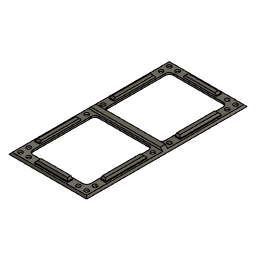
Frame Outer PLA Optimised v3 (Autodesk Fusion 360 design; units mm, degrees)
Autodesk Fusion 360 part; units mm, degrees
sketch "Sketch1" plane through (0, 0, 0) normal (0, 0, 1) x (1, 0, 0)
  line L0 (0, 0) -> (100, 0)
  line L1 (100, 0) -> (100, 200)
  line L2 (100, 200) -> (0, 200)
  line L3 (0, 200) -> (0, 0)
  line L4 (15, 15) -> (85, 15)
  line L5 (85, 15) -> (85, 185)
  line L6 (85, 185) -> (15, 185)
  line L7 (15, 185) -> (15, 15)
  dimension "d1" = 100
  dimension "d2" = 200
  dimension "d5" = 70
  dimension "d6" = 170
  dimension "d7" = 70
  constraint horizontal L0
  constraint vertical L1
  constraint horizontal L2
  constraint vertical L3
  constraint coincident L0.start L3.end
  constraint perpendicular L1 L4
  constraint perpendicular L2 L5
  constraint perpendicular L5 L6
  measures "d1" distance of L0.start L0.end
  measures "d2" distance of L0.start L2.end
  measures "d5" distance of L4.start L4.end
  measures "d6" distance of L4.end L5.end
  measures "d7" distance of L5.end L6.end
extrude "Extrude1" add sketch "Sketch1" along normal blind 5
fillet "Fillet1" radius 5 1 edges at (15, 185, 2.5)
fillet "Fillet2" radius 5 1 edges at (85, 185, 2.5)
fillet "Fillet3" radius 5 1 edges at (85, 15, 2.5)
fillet "Fillet4" radius 5 1 edges at (15, 15, 2.5)
chamfer "Chamfer1" distance 5 angle 45 1 edges at (0, 100, 5)
chamfer "Chamfer2" distance 5 angle 45 1 edges at (100, 100, 5)
chamfer "Chamfer3" distance 5 angle 45 1 edges at (50, 0, 5)
chamfer "Chamfer4" distance 5 angle 45 1 edges at (50, 200, 5)
sketch "Sketch2" plane through (0, 0, 5) normal (0, 0, 1) x (-1, 0, 0)
  line L0 (-15, -20) -> (-15, -180)
  arc A0 (-20, -185) -> (-15, -180) centre (-20, -180) ccw
  line L1 (-20, -185) -> (-80, -185)
  arc A1 (-85, -180) -> (-80, -185) centre (-80, -180) ccw
  line L2 (-85, -180) -> (-85, -20)
  arc A2 (-80, -15) -> (-85, -20) centre (-80, -20) ccw
  line L3 (-80, -15) -> (-20, -15)
  arc A3 (-15, -20) -> (-20, -15) centre (-20, -20) ccw
  line L4 (-95, -195) -> (-5, -195)
  line L5 (-5, -195) -> (-5, -5)
  line L6 (-5, -5) -> (-95, -5)
  line L7 (-95, -5) -> (-95, -195)
  line L8 (-95, -5) -> (-95, -100)
  line L9 (-95, -100) -> (-90, -100)
  line L10 (-90, -100) -> (-5, -100)
  line L11 (-85, -100) -> (-85, -105)
  line L12 (-85, -100) -> (-85, -95)
  line L13 (-85, -105) -> (-77.8443, -105)
  line L14 (-77.8443, -105) -> (-15, -105)
  line L15 (-85, -95) -> (-15, -95)
  dimension "d22" = 95
  dimension "d23" = 5
  constraint coincident L6.end L7.start
  constraint perpendicular L6 L8
  constraint perpendicular L7 L9
  constraint midpoint L5 L10.end
  constraint perpendicular L5 L10
  constraint midpoint L2 L11.start
  constraint perpendicular L10 L11
  constraint coincident L2 L12.end
  constraint perpendicular L10 L12
  constraint perpendicular L11 L13
  constraint coincident L0 L14.end
  constraint perpendicular L0 L14
  constraint coincident L0 L15.end
  constraint perpendicular L0 L15
  measures "d22" distance of L6.end L8.end
  measures "d23" distance of L11.start L11.end
extrude "Extrude2" add sketch "Sketch2" against normal blind 5 contours L0 L2 L10 L12 L15 | L0 L2 L10 L11 L13 L14
fillet "Fillet5" radius 5 1 edges at (85, 105, 2.5)
fillet "Fillet6" radius 5 1 edges at (15, 105, 2.5)
fillet "Fillet7" radius 5 1 edges at (15, 95, 2.5)
fillet "Fillet8" radius 5 1 edges at (85, 95, 2.5)
sketch "Sketch3" plane through (0, 0, 5) normal (0, 0, 1) x (-1, 0, 0)
  line L0 (-15, -110) -> (-15, -180)
  arc A0 (-20, -185) -> (-15, -180) centre (-20, -180) ccw
  line L1 (-20, -185) -> (-80, -185)
  arc A1 (-85, -180) -> (-80, -185) centre (-80, -180) ccw
  line L2 (-85, -180) -> (-85, -110)
  arc A2 (-80, -105) -> (-85, -110) centre (-80, -110) ccw
  line L3 (-80, -105) -> (-20, -105)
  arc A3 (-15, -110) -> (-20, -105) centre (-20, -110) ccw
  line L4 (-85, -90) -> (-85, -20)
  arc A4 (-80, -15) -> (-85, -20) centre (-80, -20) ccw
  line L5 (-80, -15) -> (-20, -15)
  arc A5 (-15, -20) -> (-20, -15) centre (-20, -20) ccw
  line L6 (-15, -20) -> (-15, -90)
  arc A6 (-20, -95) -> (-15, -90) centre (-20, -90) ccw
  line L7 (-20, -95) -> (-80, -95)
  arc A7 (-85, -90) -> (-80, -95) centre (-80, -90) ccw
  line L8 (-95, -195) -> (-5, -195)
  line L9 (-5, -195) -> (-5, -5)
  line L10 (-5, -5) -> (-95, -5)
  line L11 (-95, -5) -> (-95, -195)
  circle A8 centre (-10, -10) radius 2.5
  dimension "d34" = 5
  measures "d34" diameter of A8
extrude "Extrude3" cut sketch "Sketch3" against normal blind 5 contours A8
sketch "Sketch4" plane through (0, 0, 5) normal (0, 0, 1) x (-1, 0, 0)
  circle A0 centre (-10, -10) radius 2.5
  line L0 (-15, -110) -> (-15, -180)
  arc A1 (-20, -185) -> (-15, -180) centre (-20, -180) ccw
  line L1 (-20, -185) -> (-80, -185)
  arc A2 (-85, -180) -> (-80, -185) centre (-80, -180) ccw
  line L2 (-85, -180) -> (-85, -110)
  arc A3 (-80, -105) -> (-85, -110) centre (-80, -110) ccw
  line L3 (-80, -105) -> (-20, -105)
  arc A4 (-15, -110) -> (-20, -105) centre (-20, -110) ccw
  line L4 (-85, -90) -> (-85, -20)
  arc A5 (-80, -15) -> (-85, -20) centre (-80, -20) ccw
  line L5 (-80, -15) -> (-20, -15)
  arc A6 (-15, -20) -> (-20, -15) centre (-20, -20) ccw
  line L6 (-15, -20) -> (-15, -90)
  arc A7 (-20, -95) -> (-15, -90) centre (-20, -90) ccw
  line L7 (-20, -95) -> (-80, -95)
  arc A8 (-85, -90) -> (-80, -95) centre (-80, -90) ccw
  line L8 (-95, -195) -> (-5, -195)
  line L9 (-5, -195) -> (-5, -5)
  line L10 (-5, -5) -> (-95, -5)
  line L11 (-95, -5) -> (-95, -195)
  circle A9 centre (-90, -10) radius 2.5
  dimension "d37" = 5
  measures "d37" diameter of A9
extrude "Extrude4" cut sketch "Sketch4" against normal blind 5 contours A9
sketch "Sketch5" plane through (0, 0, 5) normal (0, 0, 1) x (-1, 0, 0)
  circle A0 centre (-90, -10) radius 2.5
  circle A1 centre (-10, -10) radius 2.5
  line L0 (-15, -110) -> (-15, -180)
  arc A2 (-20, -185) -> (-15, -180) centre (-20, -180) ccw
  line L1 (-20, -185) -> (-80, -185)
  arc A3 (-85, -180) -> (-80, -185) centre (-80, -180) ccw
  line L2 (-85, -180) -> (-85, -110)
  arc A4 (-80, -105) -> (-85, -110) centre (-80, -110) ccw
  line L3 (-80, -105) -> (-20, -105)
  arc A5 (-15, -110) -> (-20, -105) centre (-20, -110) ccw
  line L4 (-85, -90) -> (-85, -20)
  arc A6 (-80, -15) -> (-85, -20) centre (-80, -20) ccw
  line L5 (-80, -15) -> (-20, -15)
  arc A7 (-15, -20) -> (-20, -15) centre (-20, -20) ccw
  line L6 (-15, -20) -> (-15, -90)
  arc A8 (-20, -95) -> (-15, -90) centre (-20, -90) ccw
  line L7 (-20, -95) -> (-80, -95)
  arc A9 (-85, -90) -> (-80, -95) centre (-80, -90) ccw
  line L8 (-95, -195) -> (-5, -195)
  line L9 (-5, -195) -> (-5, -5)
  line L10 (-5, -5) -> (-95, -5)
  line L11 (-95, -5) -> (-95, -195)
  circle A10 centre (-90, -190) radius 2.5
  dimension "d40" = 5
  measures "d40" diameter of A10
extrude "Extrude5" cut sketch "Sketch5" against normal blind 5 contours A10
sketch "Sketch6" plane through (0, 0, 5) normal (0, 0, 1) x (-1, 0, 0)
  circle A0 centre (-90, -190) radius 2.5
  circle A1 centre (-90, -10) radius 2.5
  circle A2 centre (-10, -10) radius 2.5
  line L0 (-15, -110) -> (-15, -180)
  arc A3 (-20, -185) -> (-15, -180) centre (-20, -180) ccw
  line L1 (-20, -185) -> (-80, -185)
  arc A4 (-85, -180) -> (-80, -185) centre (-80, -180) ccw
  line L2 (-85, -180) -> (-85, -110)
  arc A5 (-80, -105) -> (-85, -110) centre (-80, -110) ccw
  line L3 (-80, -105) -> (-20, -105)
  arc A6 (-15, -110) -> (-20, -105) centre (-20, -110) ccw
  line L4 (-85, -90) -> (-85, -20)
  arc A7 (-80, -15) -> (-85, -20) centre (-80, -20) ccw
  line L5 (-80, -15) -> (-20, -15)
  arc A8 (-15, -20) -> (-20, -15) centre (-20, -20) ccw
  line L6 (-15, -20) -> (-15, -90)
  arc A9 (-20, -95) -> (-15, -90) centre (-20, -90) ccw
  line L7 (-20, -95) -> (-80, -95)
  arc A10 (-85, -90) -> (-80, -95) centre (-80, -90) ccw
  line L8 (-95, -195) -> (-5, -195)
  line L9 (-5, -195) -> (-5, -5)
  line L10 (-5, -5) -> (-95, -5)
  line L11 (-95, -5) -> (-95, -195)
  circle A11 centre (-10, -190) radius 2.5
  dimension "d43" = 5
  measures "d43" diameter of A11
extrude "Extrude6" cut sketch "Sketch6" against normal blind 5 contours A11
sketch "Sketch7" plane through (0, 0, 5) normal (0, 0, 1) x (-1, 0, 0)
  circle A0 centre (-10, -190) radius 2.5
  circle A1 centre (-90, -190) radius 2.5
  circle A2 centre (-90, -10) radius 2.5
  circle A3 centre (-10, -10) radius 2.5
  line L0 (-15, -110) -> (-15, -180)
  arc A4 (-20, -185) -> (-15, -180) centre (-20, -180) ccw
  line L1 (-20, -185) -> (-80, -185)
  arc A5 (-85, -180) -> (-80, -185) centre (-80, -180) ccw
  line L2 (-85, -180) -> (-85, -110)
  arc A6 (-80, -105) -> (-85, -110) centre (-80, -110) ccw
  line L3 (-80, -105) -> (-20, -105)
  arc A7 (-15, -110) -> (-20, -105) centre (-20, -110) ccw
  line L4 (-85, -90) -> (-85, -20)
  arc A8 (-80, -15) -> (-85, -20) centre (-80, -20) ccw
  line L5 (-80, -15) -> (-20, -15)
  arc A9 (-15, -20) -> (-20, -15) centre (-20, -20) ccw
  line L6 (-15, -20) -> (-15, -90)
  arc A10 (-20, -95) -> (-15, -90) centre (-20, -90) ccw
  line L7 (-20, -95) -> (-80, -95)
  arc A11 (-85, -90) -> (-80, -95) centre (-80, -90) ccw
  line L8 (-95, -195) -> (-5, -195)
  line L9 (-5, -195) -> (-5, -5)
  line L10 (-5, -5) -> (-95, -5)
  line L11 (-95, -5) -> (-95, -195)
  circle A12 centre (-90, -90) radius 2.5
  dimension "d46" = 5
  measures "d46" diameter of A12
extrude "Extrude7" cut sketch "Sketch7" against normal blind 5 contours A12
sketch "Sketch8" plane through (0, 0, 5) normal (0, 0, 1) x (-1, 0, 0)
  circle A0 centre (-90, -90) radius 2.5
  circle A1 centre (-10, -190) radius 2.5
  circle A2 centre (-90, -190) radius 2.5
  circle A3 centre (-90, -10) radius 2.5
  circle A4 centre (-10, -10) radius 2.5
  line L0 (-15, -110) -> (-15, -180)
  arc A5 (-20, -185) -> (-15, -180) centre (-20, -180) ccw
  line L1 (-20, -185) -> (-80, -185)
  arc A6 (-85, -180) -> (-80, -185) centre (-80, -180) ccw
  line L2 (-85, -180) -> (-85, -110)
  arc A7 (-80, -105) -> (-85, -110) centre (-80, -110) ccw
  line L3 (-80, -105) -> (-20, -105)
  arc A8 (-15, -110) -> (-20, -105) centre (-20, -110) ccw
  line L4 (-85, -90) -> (-85, -20)
  arc A9 (-80, -15) -> (-85, -20) centre (-80, -20) ccw
  line L5 (-80, -15) -> (-20, -15)
  arc A10 (-15, -20) -> (-20, -15) centre (-20, -20) ccw
  line L6 (-15, -20) -> (-15, -90)
  arc A11 (-20, -95) -> (-15, -90) centre (-20, -90) ccw
  line L7 (-20, -95) -> (-80, -95)
  arc A12 (-85, -90) -> (-80, -95) centre (-80, -90) ccw
  line L8 (-95, -195) -> (-5, -195)
  line L9 (-5, -195) -> (-5, -5)
  line L10 (-5, -5) -> (-95, -5)
  line L11 (-95, -5) -> (-95, -195)
  circle A13 centre (-90, -110) radius 2.5
  dimension "d49" = 5
  measures "d49" diameter of A13
extrude "Extrude8" cut sketch "Sketch8" against normal blind 5 contours A13
sketch "Sketch9" plane through (0, 0, 5) normal (0, 0, 1) x (-1, 0, 0)
  circle A0 centre (-90, -110) radius 2.5
  circle A1 centre (-90, -90) radius 2.5
  circle A2 centre (-10, -190) radius 2.5
  circle A3 centre (-90, -190) radius 2.5
  circle A4 centre (-90, -10) radius 2.5
  circle A5 centre (-10, -10) radius 2.5
  line L0 (-15, -110) -> (-15, -180)
  arc A6 (-20, -185) -> (-15, -180) centre (-20, -180) ccw
  line L1 (-20, -185) -> (-80, -185)
  arc A7 (-85, -180) -> (-80, -185) centre (-80, -180) ccw
  line L2 (-85, -180) -> (-85, -110)
  arc A8 (-80, -105) -> (-85, -110) centre (-80, -110) ccw
  line L3 (-80, -105) -> (-20, -105)
  arc A9 (-15, -110) -> (-20, -105) centre (-20, -110) ccw
  line L4 (-85, -90) -> (-85, -20)
  arc A10 (-80, -15) -> (-85, -20) centre (-80, -20) ccw
  line L5 (-80, -15) -> (-20, -15)
  arc A11 (-15, -20) -> (-20, -15) centre (-20, -20) ccw
  line L6 (-15, -20) -> (-15, -90)
  arc A12 (-20, -95) -> (-15, -90) centre (-20, -90) ccw
  line L7 (-20, -95) -> (-80, -95)
  arc A13 (-85, -90) -> (-80, -95) centre (-80, -90) ccw
  line L8 (-95, -195) -> (-5, -195)
  line L9 (-5, -195) -> (-5, -5)
  line L10 (-5, -5) -> (-95, -5)
  line L11 (-95, -5) -> (-95, -195)
  circle A14 centre (-10, -110) radius 2.5
  circle A15 centre (-10, -90) radius 2.5
  dimension "d52" = 5
  dimension "d53" = 5
  measures "d52" diameter of A14
  measures "d53" diameter of A15
extrude "Extrude9" cut sketch "Sketch9" against normal blind 5 contours A14 | A15
extrude "Extrude10" cut 1 faces at (40, 101.6667, 0) along direction (0, 0, 1) blind 3
sketch "Sketch10" plane through (0, 0, 5) normal (0, 0, 1) x (-1, 0, 0)
  circle A0 centre (-10, -90) radius 2.5
  circle A1 centre (-10, -110) radius 2.5
  circle A2 centre (-90, -110) radius 2.5
  circle A3 centre (-90, -90) radius 2.5
  circle A4 centre (-10, -190) radius 2.5
  circle A5 centre (-90, -190) radius 2.5
  circle A6 centre (-90, -10) radius 2.5
  circle A7 centre (-10, -10) radius 2.5
  line L0 (-15, -110) -> (-15, -180)
  arc A8 (-20, -185) -> (-15, -180) centre (-20, -180) ccw
  line L1 (-20, -185) -> (-80, -185)
  arc A9 (-85, -180) -> (-80, -185) centre (-80, -180) ccw
  line L2 (-85, -180) -> (-85, -110)
  arc A10 (-80, -105) -> (-85, -110) centre (-80, -110) ccw
  line L3 (-80, -105) -> (-20, -105)
  arc A11 (-15, -110) -> (-20, -105) centre (-20, -110) ccw
  line L4 (-85, -90) -> (-85, -20)
  arc A12 (-80, -15) -> (-85, -20) centre (-80, -20) ccw
  line L5 (-80, -15) -> (-20, -15)
  arc A13 (-15, -20) -> (-20, -15) centre (-20, -20) ccw
  line L6 (-15, -20) -> (-15, -90)
  arc A14 (-20, -95) -> (-15, -90) centre (-20, -90) ccw
  line L7 (-20, -95) -> (-80, -95)
  arc A15 (-85, -90) -> (-80, -95) centre (-80, -90) ccw
  line L8 (-95, -195) -> (-5, -195)
  line L9 (-5, -195) -> (-5, -5)
  line L10 (-5, -5) -> (-95, -5)
  line L11 (-95, -5) -> (-95, -195)
  line L12 (-5, -100) -> (-5, -103)
  line L13 (-5, -103) -> (-95, -103)
  line L14 (-95, -103) -> (-95, -97)
  line L15 (-95, -97) -> (-5, -97)
  line L16 (-5, -97) -> (-5, -103)
  dimension "d58" = 3
  dimension "d59" = 6
  constraint midpoint L9 L12.start
  constraint parallel L9 L12
  constraint horizontal L13
  constraint vertical L14
  constraint horizontal L15
  constraint vertical L16
  measures "d58" distance of L12.start L12.end
  measures "d59" distance of L12.end L15.end
extrude "Extrude11" add sketch "Sketch10" along normal blind 3 contours L9 L11 L12 L13 L14 L15 L16
chamfer "Chamfer5" distance 3 angle 45 1 edges at (5, 100, 8)
chamfer "Chamfer6" distance 3 angle 45 1 edges at (95, 100, 8)
sketch "Sketch11" plane through (0, 0, 5) normal (0, 0, 1) x (-1, 0, 0)
  line L0 (-85, -90) -> (-85, -20)
  arc A0 (-80, -15) -> (-85, -20) centre (-80, -20) ccw
  line L1 (-80, -15) -> (-20, -15)
  arc A1 (-15, -20) -> (-20, -15) centre (-20, -20) ccw
  line L2 (-15, -20) -> (-15, -90)
  arc A2 (-20, -95) -> (-15, -90) centre (-20, -90) ccw
  line L3 (-20, -95) -> (-80, -95)
  arc A3 (-85, -90) -> (-80, -95) centre (-80, -90) ccw
  circle A4 centre (-10, -10) radius 2.5
  circle A5 centre (-90, -10) radius 2.5
  circle A6 centre (-90, -90) radius 2.5
  circle A7 centre (-10, -90) radius 2.5
  line L4 (-95, -97) -> (-5, -97)
  line L5 (-5, -97) -> (-5, -5)
  line L6 (-5, -5) -> (-95, -5)
  line L7 (-95, -5) -> (-95, -97)
  line L8 (-10, -10) -> (-20, -10)
  circle A8 centre (-20, -10) radius 2.5
  line L9 (-90, -10) -> (-80, -10)
  circle A9 centre (-80, -10) radius 2.5
  line L10 (-90, -10) -> (-90, -20)
  circle A10 centre (-90, -20) radius 2.5
  line L11 (-10, -10) -> (-10, -20)
  circle A11 centre (-10, -20) radius 2.5
  dimension "d64" = 10
  dimension "d65" = 5
  dimension "d66" = 10
  dimension "d67" = 5
  dimension "d68" = 10
  dimension "d69" = 5
  dimension "d70" = 10
  dimension "d71" = 5
  constraint coincident A4.centre L8.start
  constraint horizontal L8
  constraint coincident L8.end A8.centre
  constraint coincident A5.centre L9.start
  constraint horizontal L9
  constraint coincident L9.end A9.centre
  constraint perpendicular L9 L10
  constraint coincident L10.end A10.centre
  constraint perpendicular L8 L11
  constraint coincident L11.end A11.centre
  measures "d64" distance of A4.centre L8.end
  measures "d65" diameter of A8
  measures "d66" distance of A5.centre L9.end
  measures "d67" diameter of A9
  measures "d68" distance of A5.centre L10.end
  measures "d69" diameter of A10
  measures "d70" distance of A4.centre L11.end
  measures "d71" diameter of A11
extrude "Extrude12" cut sketch "Sketch11" against normal blind 5 contours A8 | A9 | A10 | A11
sketch "Sketch12" plane through (0, 0, 5) normal (0, 0, 1) x (-1, 0, 0)
  circle A0 centre (-10, -110) radius 2.5
  circle A1 centre (-90, -110) radius 2.5
  circle A2 centre (-10, -190) radius 2.5
  circle A3 centre (-90, -190) radius 2.5
  line L0 (-15, -110) -> (-15, -180)
  arc A4 (-20, -185) -> (-15, -180) centre (-20, -180) ccw
  line L1 (-20, -185) -> (-80, -185)
  arc A5 (-85, -180) -> (-80, -185) centre (-80, -180) ccw
  line L2 (-85, -180) -> (-85, -110)
  arc A6 (-80, -105) -> (-85, -110) centre (-80, -110) ccw
  line L3 (-80, -105) -> (-20, -105)
  arc A7 (-15, -110) -> (-20, -105) centre (-20, -110) ccw
  line L4 (-5, -103) -> (-95, -103)
  line L5 (-95, -103) -> (-95, -195)
  line L6 (-95, -195) -> (-5, -195)
  line L7 (-5, -195) -> (-5, -103)
  line L8 (-10, -190) -> (-10, -180)
  line L9 (-10, -190) -> (-20, -190)
  circle A8 centre (-10, -180) radius 2.5
  circle A9 centre (-20, -190) radius 2.5
  line L10 (-90, -190) -> (-90, -180)
  line L11 (-90, -190) -> (-80, -190)
  circle A10 centre (-90, -180) radius 2.5
  circle A11 centre (-80, -190) radius 2.5
  dimension "d74" = 10
  dimension "d75" = 10
  dimension "d76" = 5
  dimension "d77" = 5
  dimension "d78" = 10
  dimension "d79" = 10
  dimension "d80" = 5
  dimension "d81" = 5
  constraint coincident A2.centre L8.start
  constraint vertical L8
  constraint perpendicular L8 L9
  constraint coincident L8.end A8.centre
  constraint coincident L9.end A9.centre
  constraint coincident A3.centre L10.start
  constraint vertical L10
  constraint perpendicular L10 L11
  constraint coincident L10.end A10.centre
  constraint coincident L11.end A11.centre
  measures "d74" distance of A2.centre L8.end
  measures "d75" distance of A2.centre L9.end
  measures "d76" diameter of A8
  measures "d77" diameter of A9
  measures "d78" distance of A3.centre L10.end
  measures "d79" distance of A3.centre L11.end
  measures "d80" diameter of A10
  measures "d81" diameter of A11
extrude "Extrude13" cut sketch "Sketch12" against normal blind 5 contours A8 | A9 | A10 | A11
sketch "Sketch13" plane through (0, 0, 5) normal (0, 0, 1) x (-1, 0, 0)
  circle A0 centre (-90, -180) radius 2.5
  circle A1 centre (-20, -190) radius 2.5
  circle A2 centre (-80, -190) radius 2.5
  circle A3 centre (-10, -180) radius 2.5
  circle A4 centre (-10, -110) radius 2.5
  circle A5 centre (-90, -110) radius 2.5
  circle A6 centre (-10, -190) radius 2.5
  circle A7 centre (-90, -190) radius 2.5
  line L0 (-15, -110) -> (-15, -180)
  arc A8 (-20, -185) -> (-15, -180) centre (-20, -180) ccw
  line L1 (-20, -185) -> (-80, -185)
  arc A9 (-85, -180) -> (-80, -185) centre (-80, -180) ccw
  line L2 (-85, -180) -> (-85, -110)
  arc A10 (-80, -105) -> (-85, -110) centre (-80, -110) ccw
  line L3 (-80, -105) -> (-20, -105)
  arc A11 (-15, -110) -> (-20, -105) centre (-20, -110) ccw
  line L4 (-5, -103) -> (-95, -103)
  line L5 (-95, -103) -> (-95, -195)
  line L6 (-95, -195) -> (-5, -195)
  line L7 (-5, -195) -> (-5, -103)
  line L8 (-10, -20) -> (-10, -30)
  line L9 (-10, -90) -> (-10, -80)
  line L10 (-10, -80) -> (-7, -80)
  line L11 (-7, -80) -> (-13, -80)
  line L12 (-13, -80) -> (-13, -30)
  line L13 (-13, -30) -> (-7, -30)
  line L14 (-7, -30) -> (-7, -80)
  dimension "d84" = 10
  dimension "d85" = 10
  dimension "d86" = 3
  dimension "d87" = 6
  constraint vertical L8
  constraint vertical L9
  constraint perpendicular L9 L10
  constraint horizontal L11
  constraint vertical L12
  constraint horizontal L13
  constraint vertical L14
  measures "d84" distance of L8.start L8.end
  measures "d85" distance of L9.start L9.end
  measures "d86" distance of L9.end L10.end
  measures "d87" distance of L10.end L11.end
extrude "Extrude14" add sketch "Sketch13" along normal blind 3 contours L10 L11 L12 L13 L14
chamfer "Chamfer7" distance 2 angle 45 1 edges at (7, 55, 8)
sketch "Sketch14" plane through (0, 0, 5) normal (0, 0, 1) x (-1, 0, 0)
  line L0 (-7, -30) -> (-7, -80)
  line L1 (-7, -80) -> (-13, -80)
  line L2 (-13, -80) -> (-13, -30)
  line L3 (-13, -30) -> (-7, -30)
  circle A0 centre (-10, -20) radius 2.5
  circle A1 centre (-80, -10) radius 2.5
  circle A2 centre (-20, -10) radius 2.5
  circle A3 centre (-90, -20) radius 2.5
  line L4 (-85, -90) -> (-85, -20)
  arc A4 (-80, -15) -> (-85, -20) centre (-80, -20) ccw
  line L5 (-80, -15) -> (-20, -15)
  arc A5 (-15, -20) -> (-20, -15) centre (-20, -20) ccw
  line L6 (-15, -20) -> (-15, -90)
  arc A6 (-20, -95) -> (-15, -90) centre (-20, -90) ccw
  line L7 (-20, -95) -> (-80, -95)
  arc A7 (-85, -90) -> (-80, -95) centre (-80, -90) ccw
  circle A8 centre (-10, -10) radius 2.5
  circle A9 centre (-90, -10) radius 2.5
  circle A10 centre (-90, -90) radius 2.5
  circle A11 centre (-10, -90) radius 2.5
  line L8 (-95, -97) -> (-5, -97)
  line L9 (-5, -97) -> (-5, -5)
  line L10 (-5, -5) -> (-95, -5)
  line L11 (-95, -5) -> (-95, -97)
  line L12 (-20, -10) -> (-30, -10)
  line L13 (-80, -10) -> (-70, -10)
  line L14 (-30, -10) -> (-30, -13)
  line L15 (-70, -10) -> (-70, -7)
  line L16 (-30, -13) -> (-70, -13)
  line L17 (-70, -13) -> (-70, -7)
  line L18 (-70, -7) -> (-30, -7)
  line L19 (-30, -7) -> (-30, -13)
  dimension "d91" = 10
  dimension "d92" = 10
  dimension "d93" = 3
  dimension "d94" = 3
  constraint coincident A2.centre L12.start
  constraint horizontal L12
  constraint coincident A1.centre L13.start
  constraint horizontal L13
  constraint perpendicular L12 L14
  constraint perpendicular L13 L15
  constraint horizontal L16
  constraint vertical L17
  constraint horizontal L18
  constraint vertical L19
  measures "d91" distance of A2.centre L12.end
  measures "d92" distance of A1.centre L13.end
  measures "d93" distance of L12.end L14.end
  measures "d94" distance of L13.end L15.end
extrude "Extrude15" add sketch "Sketch14" along normal blind 5 contours L14 L15 L16 L17 L18 L19
extrude "Extrude16" cut 1 faces at (56.6667, 11, 10) along direction (0, 0, -1) blind 2
chamfer "Chamfer8" distance 2 angle 45 1 edges at (50, 7, 8)
chamfer "Chamfer9" distance 2 angle 45 1 edges at (30, 11, 8)
chamfer "Chamfer10" distance 2 angle 45 1 edges at (70, 11, 8)
chamfer "Chamfer11" distance 2 angle 45 1 edges at (11, 30, 8)
chamfer "Chamfer12" distance 2 angle 45 1 edges at (11, 80, 8)
sketch "Sketch15" plane through (0, 0, 5) normal (0, 0, 1) x (-1, 0, 0)
  line L0 (-30, -7) -> (-30, -13)
  line L1 (-30, -13) -> (-70, -13)
  line L2 (-70, -13) -> (-70, -7)
  line L3 (-70, -7) -> (-30, -7)
  line L4 (-7, -30) -> (-7, -80)
  line L5 (-7, -80) -> (-13, -80)
  line L6 (-13, -80) -> (-13, -30)
  line L7 (-13, -30) -> (-7, -30)
  circle A0 centre (-10, -20) radius 2.5
  circle A1 centre (-80, -10) radius 2.5
  circle A2 centre (-20, -10) radius 2.5
  circle A3 centre (-90, -20) radius 2.5
  line L8 (-85, -90) -> (-85, -20)
  arc A4 (-80, -15) -> (-85, -20) centre (-80, -20) ccw
  line L9 (-80, -15) -> (-20, -15)
  arc A5 (-15, -20) -> (-20, -15) centre (-20, -20) ccw
  line L10 (-15, -20) -> (-15, -90)
  arc A6 (-20, -95) -> (-15, -90) centre (-20, -90) ccw
  line L11 (-20, -95) -> (-80, -95)
  arc A7 (-85, -90) -> (-80, -95) centre (-80, -90) ccw
  circle A8 centre (-10, -10) radius 2.5
  circle A9 centre (-90, -10) radius 2.5
  circle A10 centre (-90, -90) radius 2.5
  circle A11 centre (-10, -90) radius 2.5
  line L12 (-95, -97) -> (-5, -97)
  line L13 (-5, -97) -> (-5, -5)
  line L14 (-5, -5) -> (-95, -5)
  line L15 (-95, -5) -> (-95, -97)
  line L16 (-90, -20) -> (-90, -30)
  line L17 (-90, -90) -> (-90, -80)
  line L18 (-90, -80) -> (-87, -80)
  line L19 (-90, -30) -> (-93, -30)
  line L20 (-87, -80) -> (-93, -80)
  line L21 (-93, -80) -> (-93, -30)
  line L22 (-93, -30) -> (-87, -30)
  line L23 (-87, -30) -> (-87, -80)
  dimension "d104" = 10
  dimension "d105" = 10
  dimension "d106" = 3
  dimension "d107" = 3
  constraint coincident A3.centre L16.start
  constraint parallel L8 L16
  constraint coincident A10.centre L17.start
  constraint parallel L8 L17
  constraint perpendicular L17 L18
  constraint perpendicular L16 L19
  constraint horizontal L20
  constraint vertical L21
  constraint horizontal L22
  constraint vertical L23
  measures "d104" distance of A3.centre L16.end
  measures "d105" distance of A10.centre L17.end
  measures "d106" distance of L17.end L18.end
  measures "d107" distance of L16.end L19.end
extrude "Extrude17" add sketch "Sketch15" along normal blind 3 contours L18 L19 L20 L21 L22 L23
chamfer "Chamfer13" distance 2 angle 45 1 edges at (93, 55, 8)
chamfer "Chamfer14" distance 2 angle 45 1 edges at (89, 30, 8)
chamfer "Chamfer15" distance 2 angle 45 1 edges at (89, 80, 8)
sketch "Sketch16" plane through (0, 0, 5) normal (0, 0, 1) x (-1, 0, 0)
  circle A0 centre (-90, -180) radius 2.5
  circle A1 centre (-20, -190) radius 2.5
  circle A2 centre (-80, -190) radius 2.5
  circle A3 centre (-10, -180) radius 2.5
  circle A4 centre (-10, -110) radius 2.5
  circle A5 centre (-90, -110) radius 2.5
  circle A6 centre (-10, -190) radius 2.5
  circle A7 centre (-90, -190) radius 2.5
  line L0 (-15, -110) -> (-15, -180)
  arc A8 (-20, -185) -> (-15, -180) centre (-20, -180) ccw
  line L1 (-20, -185) -> (-80, -185)
  arc A9 (-85, -180) -> (-80, -185) centre (-80, -180) ccw
  line L2 (-85, -180) -> (-85, -110)
  arc A10 (-80, -105) -> (-85, -110) centre (-80, -110) ccw
  line L3 (-80, -105) -> (-20, -105)
  arc A11 (-15, -110) -> (-20, -105) centre (-20, -110) ccw
  line L4 (-5, -103) -> (-95, -103)
  line L5 (-95, -103) -> (-95, -195)
  line L6 (-95, -195) -> (-5, -195)
  line L7 (-5, -195) -> (-5, -103)
  line L8 (-90, -110) -> (-90, -120)
  line L9 (-90, -180) -> (-90, -170)
  line L10 (-80, -190) -> (-70, -190)
  line L11 (-20, -190) -> (-30, -190)
  line L12 (-10, -180) -> (-10, -170)
  line L13 (-10, -110) -> (-10, -120)
  line L14 (-90, -120) -> (-93, -120)
  line L15 (-90, -170) -> (-87, -170)
  line L16 (-70, -190) -> (-70, -187)
  line L17 (-30, -190) -> (-30, -193)
  line L18 (-10, -170) -> (-7, -170)
  line L19 (-10, -120) -> (-13, -120)
  line L20 (-7, -170) -> (-13, -170)
  line L21 (-13, -170) -> (-13, -120)
  line L22 (-13, -120) -> (-7, -120)
  line L23 (-7, -120) -> (-7, -170)
  line L24 (-30, -193) -> (-70, -193)
  line L25 (-70, -193) -> (-70, -187)
  line L26 (-70, -187) -> (-30, -187)
  line L27 (-30, -187) -> (-30, -193)
  line L28 (-87, -170) -> (-93, -170)
  line L29 (-93, -170) -> (-93, -120)
  line L30 (-93, -120) -> (-87, -120)
  line L31 (-87, -120) -> (-87, -170)
  dimension "d113" = 10
  dimension "d114" = 10
  dimension "d115" = 10
  dimension "d116" = 10
  dimension "d117" = 10
  dimension "d118" = 10
  dimension "d119" = 3
  dimension "d120" = 3
  dimension "d121" = 3
  dimension "d122" = 3
  dimension "d123" = 3
  dimension "d124" = 3
  constraint coincident A5.centre L8.start
  constraint vertical L8
  constraint coincident A0.centre L9.start
  constraint parallel L2 L9
  constraint coincident A2.centre L10.start
  constraint parallel L1 L10
  constraint coincident A1.centre L11.start
  constraint horizontal L11
  constraint coincident A3.centre L12.start
  constraint vertical L12
  constraint coincident A4.centre L13.start
  constraint perpendicular L4 L13
  constraint perpendicular L8 L14
  constraint perpendicular L9 L15
  constraint perpendicular L10 L16
  constraint perpendicular L11 L17
  constraint perpendicular L12 L18
  constraint perpendicular L13 L19
  constraint horizontal L20
  constraint vertical L21
  constraint horizontal L22
  constraint vertical L23
  constraint horizontal L24
  constraint vertical L25
  constraint horizontal L26
  constraint vertical L27
  constraint horizontal L28
  constraint vertical L29
  constraint horizontal L30
  constraint vertical L31
  measures "d113" distance of A5.centre L8.end
  measures "d114" distance of A0.centre L9.end
  measures "d115" distance of A2.centre L10.end
  measures "d116" distance of A1.centre L11.end
  measures "d117" distance of A3.centre L12.end
  measures "d118" distance of A4.centre L13.end
  measures "d119" distance of L8.end L14.end
  measures "d120" distance of L9.end L15.end
  measures "d121" distance of L10.end L16.end
  measures "d122" distance of L11.end L17.end
  measures "d123" distance of L12.end L18.end
  measures "d124" distance of L13.end L19.end
extrude "Extrude18" add sketch "Sketch16" along normal blind 3 contours L14 L15 L28 L29 L30 L31 | L16 L17 L24 L25 L26 L27 | L18 L19 L20 L21 L22 L23
chamfer "Chamfer16" distance 2 angle 45 1 edges at (93, 145, 8)
chamfer "Chamfer17" distance 2 angle 45 1 edges at (89, 170, 8)
chamfer "Chamfer18" distance 2 angle 45 1 edges at (70, 190, 8)
chamfer "Chamfer19" distance 2 angle 45 1 edges at (49, 193, 8)
chamfer "Chamfer20" distance 2 angle 45 1 edges at (10, 170, 8)
chamfer "Chamfer21" distance 2 angle 45 1 edges at (89, 120, 8)
chamfer "Chamfer22" distance 2 angle 45 1 edges at (10, 120, 8)
chamfer "Chamfer23" distance 2 angle 45 1 edges at (7, 145, 8)
chamfer "Chamfer24" distance 2 angle 45 1 edges at (30, 189, 8)
equation "d41 = 0.00 mm - 5 mm"
